Autodesk Fusion 360 part; units mm, degrees
(part 2 of 2)
sketch "Sketch26" plane through (0, 0, 10) normal (0, 0, 1) x (-1, 0, 0)
  circle A0 centre (11.42, 31.75) radius 0.762
  circle A1 centre (20.71, -12.7) radius 0.762
  circle A2 centre (23.25, 2.54) radius 0.762
  circle A3 centre (20.71, 20.32) radius 0.762
  circle A4 centre (13.96, 6.35) radius 0.762
  circle A5 centre (11.42, -13.97) radius 0.762
  circle A6 centre (8.88, -16.51) radius 0.762
  circle A7 centre (3.8, -31.75) radius 0.762
  circle A8 centre (23.25, -2.54) radius 0.762
  circle A9 centre (6.34, -34.29) radius 0.762
  circle A10 centre (3.8, -26.67) radius 0.762
  circle A11 centre (6.34, -24.13) radius 0.762
  circle A12 centre (20.71, -30.48) radius 0.762
  circle A13 centre (3.8, 3.81) radius 0.762
  circle A14 centre (3.8, 21.59) radius 0.762
  circle A15 centre (23.25, 30.48) radius 0.762
  circle A16 centre (13.96, -31.75) radius 0.762
  circle A17 centre (8.88, 19.05) radius 0.762
  circle A18 centre (11.42, 29.21) radius 0.762
  circle A19 centre (11.42, -29.21) radius 0.762
  circle A20 centre (11.42, 1.27) radius 0.762
  circle A21 centre (11.42, 3.81) radius 0.762
  circle A22 centre (3.8, -24.13) radius 0.762
  circle A23 centre (20.71, 33.02) radius 0.762
  circle A24 centre (20.71, 30.48) radius 0.762
  circle A25 centre (8.88, 21.59) radius 0.762
  circle A26 centre (6.34, -36.83) radius 0.762
  circle A27 centre (3.8, 24.13) radius 0.762
  circle A28 centre (23.25, 12.7) radius 0.762
  circle A29 centre (6.34, 26.67) radius 0.762
  circle A30 centre (13.96, 36.83) radius 0.762
  circle A31 centre (13.96, -36.83) radius 0.762
  circle A32 centre (13.96, -8.89) radius 0.762
  circle A33 centre (23.25, 0) radius 0.762
  circle A34 centre (3.8, -13.97) radius 0.762
  circle A35 centre (6.34, -6.35) radius 0.762
  circle A36 centre (11.42, -16.51) radius 0.762
  circle A37 centre (13.96, 16.51) radius 0.762
  circle A38 centre (20.71, 15.24) radius 0.762
  circle A39 centre (11.42, -19.05) radius 0.762
  circle A40 centre (20.71, -5.08) radius 0.762
  circle A41 centre (6.34, 36.83) radius 0.762
  circle A42 centre (6.34, -31.75) radius 0.762
  circle A43 centre (3.8, -21.59) radius 0.762
  circle A44 centre (13.96, 11.43) radius 0.762
  circle A45 centre (8.88, 3.81) radius 0.762
  circle A46 centre (13.96, -1.27) radius 0.762
  circle A47 centre (11.42, -34.29) radius 0.762
  circle A48 centre (23.25, -35.56) radius 0.762
  circle A49 centre (8.88, 36.83) radius 0.762
  circle A50 centre (11.42, -11.43) radius 0.762
  circle A51 centre (6.34, 8.89) radius 0.762
  circle A52 centre (3.8, -29.21) radius 0.762
  circle A53 centre (3.8, 29.21) radius 0.762
  circle A54 centre (6.34, 6.35) radius 0.762
  circle A55 centre (11.42, -1.27) radius 0.762
  circle A56 centre (6.34, 34.29) radius 0.762
  circle A57 centre (6.34, -8.89) radius 0.762
  circle A58 centre (6.34, 31.75) radius 0.762
  circle A59 centre (13.96, 13.97) radius 0.762
  circle A60 centre (8.88, 8.89) radius 0.762
  circle A61 centre (8.88, -36.83) radius 0.762
  circle A62 centre (8.88, -11.43) radius 0.762
  circle A63 centre (13.96, -29.21) radius 0.762
  circle A64 centre (20.71, 35.56) radius 0.762
  circle A65 centre (11.42, -31.75) radius 0.762
  circle A66 centre (8.88, -1.27) radius 0.762
  circle A67 centre (8.88, 13.97) radius 0.762
  circle A68 centre (23.25, 27.94) radius 0.762
  circle A69 centre (13.96, 31.75) radius 0.762
  circle A70 centre (6.34, -16.51) radius 0.762
  circle A71 centre (13.96, 26.67) radius 0.762
  circle A72 centre (6.34, -1.27) radius 0.762
  circle A73 centre (11.42, -8.89) radius 0.762
  circle A74 centre (6.34, -19.05) radius 0.762
  circle A75 centre (11.42, -3.81) radius 0.762
  circle A76 centre (8.88, 6.35) radius 0.762
  circle A77 centre (23.25, -30.48) radius 0.762
  circle A78 centre (23.25, -27.94) radius 0.762
  circle A79 centre (3.8, -3.81) radius 0.762
  circle A80 centre (11.42, 21.59) radius 0.762
  circle A81 centre (20.71, -20.32) radius 0.762
  circle A82 centre (3.8, -6.35) radius 0.762
  circle A83 centre (6.34, -3.81) radius 0.762
  circle A84 centre (13.96, -3.81) radius 0.762
  circle A85 centre (20.71, -2.54) radius 0.762
  circle A86 centre (6.34, -11.43) radius 0.762
  circle A87 centre (3.8, -16.51) radius 0.762
  circle A88 centre (23.25, 15.24) radius 0.762
  circle A89 centre (11.42, 16.51) radius 0.762
  circle A90 centre (6.34, -13.97) radius 0.762
  circle A91 centre (23.25, -10.16) radius 0.762
  circle A92 centre (3.8, 36.83) radius 0.762
  circle A93 centre (3.8, 34.29) radius 0.762
  circle A94 centre (13.96, 24.13) radius 0.762
  circle A95 centre (8.88, 29.21) radius 0.762
  circle A96 centre (11.42, 13.97) radius 0.762
  circle A97 centre (8.88, -3.81) radius 0.762
  circle A98 centre (23.25, 20.32) radius 0.762
  circle A99 centre (23.25, -33.02) radius 0.762
  circle A100 centre (23.25, -20.32) radius 0.762
  circle A101 centre (3.8, -8.89) radius 0.762
  circle A102 centre (11.42, 19.05) radius 0.762
  circle A103 centre (11.42, 26.67) radius 0.762
  circle A104 centre (20.71, 5.08) radius 0.762
  circle A105 centre (3.8, 19.05) radius 0.762
  circle A106 centre (13.96, -26.67) radius 0.762
  circle A107 centre (11.42, -6.35) radius 0.762
  circle A108 centre (8.88, -34.29) radius 0.762
  circle A109 centre (3.8, 13.97) radius 0.762
  circle A110 centre (6.34, -29.21) radius 0.762
  circle A111 centre (23.25, -5.08) radius 0.762
  circle A112 centre (20.71, 17.78) radius 0.762
  circle A113 centre (23.25, 10.16) radius 0.762
  circle A114 centre (11.42, -21.59) radius 0.762
  circle A115 centre (20.71, -17.78) radius 0.762
  circle A116 centre (11.42, -36.83) radius 0.762
  circle A117 centre (6.34, 19.05) radius 0.762
  circle A118 centre (3.8, -36.83) radius 0.762
  circle A119 centre (20.71, -25.4) radius 0.762
  circle A120 centre (3.8, 6.35) radius 0.762
  circle A121 centre (20.71, -33.02) radius 0.762
  circle A122 centre (13.96, -21.59) radius 0.762
  circle A123 centre (3.8, 1.27) radius 0.762
  circle A124 centre (6.34, 13.97) radius 0.762
  circle A125 centre (11.42, 34.29) radius 0.762
  circle A126 centre (3.8, 11.43) radius 0.762
  circle A127 centre (13.96, -34.29) radius 0.762
  circle A128 centre (8.88, 1.27) radius 0.762
  circle A129 centre (23.25, -17.78) radius 0.762
  circle A130 centre (23.25, 25.4) radius 0.762
  circle A131 centre (13.96, 29.21) radius 0.762
  circle A132 centre (8.88, 16.51) radius 0.762
  circle A133 centre (8.88, -31.75) radius 0.762
  circle A134 centre (13.96, -16.51) radius 0.762
  circle A135 centre (13.96, -11.43) radius 0.762
  circle A136 centre (8.88, 11.43) radius 0.762
  circle A137 centre (8.88, -24.13) radius 0.762
  circle A138 centre (3.8, 8.89) radius 0.762
  circle A139 centre (6.34, 3.81) radius 0.762
  circle A140 centre (20.71, -10.16) radius 0.762
  circle A141 centre (8.88, -19.05) radius 0.762
  circle A142 centre (3.8, -19.05) radius 0.762
  circle A143 centre (13.96, -24.13) radius 0.762
  circle A144 centre (8.88, -26.67) radius 0.762
  circle A145 centre (11.42, -24.13) radius 0.762
  circle A146 centre (13.96, 19.05) radius 0.762
  circle A147 centre (8.88, 34.29) radius 0.762
  circle A148 centre (6.34, -26.67) radius 0.762
  circle A149 centre (8.88, 31.75) radius 0.762
  circle A150 centre (13.96, 1.27) radius 0.762
  circle A151 centre (8.88, -21.59) radius 0.762
  circle A152 centre (13.96, 8.89) radius 0.762
  circle A153 centre (20.71, 25.4) radius 0.762
  circle A154 centre (23.25, -25.4) radius 0.762
  circle A155 centre (8.88, -8.89) radius 0.762
  circle A156 centre (3.8, 16.51) radius 0.762
  circle A157 centre (11.42, 11.43) radius 0.762
  circle A158 centre (20.71, 2.54) radius 0.762
  circle A159 centre (20.71, 10.16) radius 0.762
  circle A160 centre (23.25, -12.7) radius 0.762
  circle A161 centre (3.8, -11.43) radius 0.762
  circle A162 centre (8.88, 24.13) radius 0.762
  circle A163 centre (8.88, 26.67) radius 0.762
  circle A164 centre (8.88, -13.97) radius 0.762
  circle A165 centre (23.25, 17.78) radius 0.762
  circle A166 centre (3.8, -34.29) radius 0.762
  circle A167 centre (11.42, 36.83) radius 0.762
  circle A168 centre (20.71, -15.24) radius 0.762
  circle A169 centre (23.25, 5.08) radius 0.762
  circle A170 centre (11.42, -26.67) radius 0.762
  circle A171 centre (20.71, 12.7) radius 0.762
  circle A172 centre (13.96, -6.35) radius 0.762
  circle A173 centre (20.71, 27.94) radius 0.762
  circle A174 centre (8.88, -6.35) radius 0.762
  circle A175 centre (11.42, 24.13) radius 0.762
  circle A176 centre (8.88, -29.21) radius 0.762
  circle A177 centre (6.34, 24.13) radius 0.762
  circle A178 centre (6.34, 21.59) radius 0.762
  circle A179 centre (13.96, 21.59) radius 0.762
  circle A180 centre (3.8, 26.67) radius 0.762
  circle A181 centre (23.25, 35.56) radius 0.762
  circle A182 centre (20.71, 0) radius 0.762
  circle A183 centre (23.25, 33.02) radius 0.762
  circle A184 centre (6.34, -21.59) radius 0.762
  circle A185 centre (6.34, 29.21) radius 0.762
  circle A186 centre (11.42, 6.35) radius 0.762
  circle A187 centre (20.71, -35.56) radius 0.762
  circle A188 centre (11.42, 8.89) radius 0.762
  circle A189 centre (3.8, -1.27) radius 0.762
  circle A190 centre (6.34, 11.43) radius 0.762
  circle A191 centre (6.34, 1.27) radius 0.762
  circle A192 centre (20.71, -27.94) radius 0.762
  circle A193 centre (6.34, 16.51) radius 0.762
  circle A194 centre (13.96, -19.05) radius 0.762
  circle A195 centre (13.96, 34.29) radius 0.762
  circle A196 centre (23.25, -15.24) radius 0.762
  circle A197 centre (3.8, 31.75) radius 0.762
  circle A198 centre (13.96, -13.97) radius 0.762
  circle A199 centre (13.96, 3.81) radius 0.762
  line L0 (1.9, -40.715) -> (26.8, -40.715)
  line L1 (26.8, -40.715) -> (26.8, 40.715)
  line L2 (26.8, 40.715) -> (1.9, 40.715)
  line L3 (1.9, 40.715) -> (1.9, -40.715)
  line L4 (3.1037, 23.115) -> (-2.8963, 23.115)
  line L5 (-2.8963, 23.115) -> (-2.8963, 38.115)
  line L6 (-2.8963, 38.115) -> (3.1037, 38.115)
  line L7 (3.1037, 38.115) -> (3.1037, 23.115)
  line L8 (3.1037, 31.115) -> (-2.8963, 31.115)
  line L9 (3.1037, 30.115) -> (-2.8963, 30.115)
  line L10 (3.1037, 38.115) -> (-2.8963, 31.115) construction
  line L11 (-2.8963, 38.115) -> (3.1037, 31.115) construction
  line L12 (3.1037, 30.115) -> (-2.8963, 23.115) construction
  line L13 (-2.8963, 30.115) -> (3.1037, 23.115) construction
  circle A200 centre (0.1037, 34.615) radius 1.75
  circle A201 centre (0.1037, 26.615) radius 1.75
  line L14 (-1.5, 41.115) -> (1.5, 41.115)
  line L15 (1.5, 41.115) -> (1.5, 38.115) construction
  line L16 (1.5, 38.115) -> (-1.2925, 38.115) construction
  line L17 (-1.2925, 38.115) -> (-1.5, 41.115) construction
  dimension "d222" = 3.5
  dimension "d223" = 6
  dimension "d225" = 15
  dimension "d226" = 1
  dimension "d227" = 3
  constraint horizontal L4
  constraint vertical L5
  constraint horizontal L6
  constraint vertical L7
  constraint coincident L7 L8.start
  constraint coincident L5 L8.end
  constraint perpendicular L5 L8
  constraint coincident L7 L9.start
  constraint coincident L5 L9.end
  constraint perpendicular L5 L9
  constraint parallel L10 L12
  constraint midpoint L11 A200.centre
  constraint midpoint L13 A201.centre
  constraint equal A200 A201
  constraint coincident L14.end L15.start
  constraint perpendicular L14 L15
  constraint perpendicular L15 L16
  constraint coincident L14.start L17.end
  constraint midpoint L6 L16
  measures "d222" diameter of A201
  measures "d223" distance of L4.start L4.end
  measures "d225" distance of L4.start L6.end
  measures "d226" distance of L8 L9
  measures "d227" distance of L14 L16
extrude "Extrude19" add sketch "Sketch26" along normal blind 3.5 separate body contours A27 L7 | A27 A53 A180 L3 L4 L7 L9 | A180 L7 | L3 L4 L5 L9 | A53 L7 | L3 L5 L6 L8 | A92 A93 A197 L3 L6 L7 L8 | A197 L7 | A92 L7 | A93 L7 picked at (3.0916, 24.1999) picked at (3.0916, 26.7399) picked at (3.0916, 29.2799) picked at (3.0916, 31.8199) picked at (3.0916, 36.8999) picked at (3.0916, 34.3599) makes body 3 at (-1.7482, -34.0165, 12.3333) makes body 4 at (-1.845, -26.4408, 12.3333)
extrude "Extrude20" add sketch "Sketch26" along normal blind 5 contours A200 | A201 bodies 1 3 4
ref_plane "WorkPlane5" through (-0.1037, -26.615, 15.6) normal (0, 0, 1) x (-1, 0, 0)
sketch "Sketch27" plane through (0, 0, 15.6) normal (0, 0, 1) x (1, 0, 0)
  circle A0 centre (-0.1037, -26.615) radius 1.75
  circle A1 centre (-0.1037, -34.615) radius 1.75
  circle A2 centre (-0.1037, -34.615) radius 3.5
  circle A3 centre (-0.1037, -26.615) radius 3.5
  circle A4 centre (-0.1037, -34.615) radius 2.5
  circle A5 centre (-0.1037, -26.615) radius 2.5
  dimension "d228" = 7
  dimension "d231" = 0.75
  dimension "d232" = 0.75
  constraint concentric A1 A2
  constraint concentric A0 A3
  constraint equal A2 A3
  constraint concentric A1 A4
  constraint concentric A0 A5
  measures "d228" diameter of A3
  measures "d231" distance of A0 A5
  measures "d232" distance of A1 A4
extrude "Extrude21" cut sketch "Sketch27" along normal up to surface (6.7 mm away) contours A0 | A1 | A2 | A3 | A4 | A5 bodies 2
extrude "Extrude22" add sketch "Sketch27" along normal blind 8 separate body contours A0 | A1 | A4 | A5 makes body 5 at (2.3932, -34.7396, 20.9333) makes body 6 at (2.3932, -26.7396, 20.9333)
extrude "Extrude23" add sketch "Sketch27" along normal mid plane 0.8 from surface at 5.2 contours A2 | A3 bodies 2 5 6
sketch "case_floor" plane through (0, 0, 0) normal (0, 0, -1) x (1, 0, 0)
  line L0 (27.8, -41.715) -> (-29.3, -41.715)
  line L1 (-29.3, -41.715) -> (-29.3, 43.215)
  line L2 (-29.3, 43.215) -> (27.8, 43.215)
  line L3 (27.8, 43.215) -> (27.8, -41.715)
  line L4 (-32.3, -44.715) -> (30.8, -44.715)
  line L5 (30.8, -44.715) -> (30.8, 46.215)
  line L6 (30.8, 46.215) -> (-32.3, 46.215)
  line L7 (-32.3, 46.215) -> (-32.3, -44.715)
  line L8 (27.8, 43.215) -> (30.8, 43.215) construction
  line L9 (-29.3, 43.215) -> (-32.3, 43.215) construction
  line L10 (-29.3, -41.715) -> (-32.3, -41.715) construction
  line L11 (27.8, -41.715) -> (30.8, -41.715) construction
  circle A0 centre (33.8, 37.215) radius 6
  circle A1 centre (-35.3, 37.215) radius 6
  circle A2 centre (-35.3, -35.715) radius 6
  circle A3 centre (33.8, -35.715) radius 6
  circle A4 centre (33.8, 37.215) radius 1.65
  circle A5 centre (33.8, 37.215) radius 1.35
  circle A6 centre (33.8, -35.715) radius 1.65
  circle A7 centre (33.8, -35.715) radius 1.35
  circle A8 centre (-35.3, -35.715) radius 1.65
  circle A9 centre (-35.3, -35.715) radius 1.35
  circle A10 centre (-35.3, 37.215) radius 1.65
  circle A11 centre (-35.3, 37.215) radius 1.35
  dimension "d238" = 12
  dimension "d239" = 2.7
  dimension "d240" = 3.3
  constraint coincident L2.end L3.start
  constraint coincident L5 L8.end
  constraint perpendicular L5 L8
  constraint coincident L1.end L2.start
  constraint coincident L7 L9.end
  constraint perpendicular L7 L9
  constraint coincident L0.end L1.start
  constraint coincident L7 L10.end
  constraint perpendicular L7 L10
  constraint coincident L0.start L3.end
  constraint coincident L5 L11.end
  constraint perpendicular L5 L11
  constraint tangent L8 A0
  constraint tangent L3 A0
  constraint tangent L1 A1
  constraint tangent L9 A1
  constraint tangent L10 A2
  constraint tangent L1 A2
  constraint tangent L11 A3
  constraint tangent L3 A3
  constraint equal A0 A3
  constraint equal A2 A3
  constraint equal A1 A2
  constraint concentric A0 A4
  constraint concentric A4 A5
  constraint concentric A3 A6
  constraint concentric A3 A7
  constraint concentric A2 A8
  constraint concentric A8 A9
  constraint concentric A1 A10
  constraint concentric A1 A11
  constraint equal A7 A9
  constraint equal A5 A7
  constraint equal A5 A11
  constraint equal A4 A10
  constraint equal A4 A6
  constraint equal A6 A8
  measures "d238" diameter of A3
  measures "d239" diameter of A5
  measures "d240" diameter of A4
extrude "Extrude5" add sketch "case_floor" along normal blind 3 separate body contours L0 L1 L3 L4 L5 L7 A2 A3 | L0 L1 L2 L3 | L3 L5 A0 A3 | L5 A3 | L1 L7 A1 A2 | L7 A2 | L1 L2 L3 L5 L6 L7 A0 A1 | L5 A0 | L5 A3 | L7 A1 | L7 A2 | L5 A0 | L7 A1 makes body 7
extrude "Extrude17" add sketch "case_floor" against normal blind 7.6 contours L5 A3 | L7 A2 | L5 A0 | L7 A1 | A4 | A6 | A8 | A10 picked at (31.25, -35.715) picked at (-32.75, -35.715) picked at (31.25, 37.215) picked at (-32.75, 37.215) bodies 2
sketch "boss" plane through (0, 0, 7.6) normal (0, 0, 1) x (-1, 0, 0)
  circle A0 centre (-33.8, 37.215) radius 1.35
  arc A1 (-30.8, 42.4112) -> (-30.8, 32.0188) centre (-33.8, 37.215) ccw
  line L0 (-30.8, 32.0188) -> (-30.8, 42.4112)
  circle A2 centre (35.3, 37.215) radius 1.35
  arc A3 (32.3, 32.0188) -> (32.3, 42.4112) centre (35.3, 37.215) ccw
  line L1 (32.3, 42.4112) -> (32.3, 32.0188)
  circle A4 centre (-33.8, -35.715) radius 1.35
  arc A5 (-30.8, -30.5188) -> (-30.8, -40.9112) centre (-33.8, -35.715) ccw
  line L2 (-30.8, -40.9112) -> (-30.8, -30.5188)
  circle A6 centre (35.3, -35.715) radius 1.35
  arc A7 (32.3, -40.9112) -> (32.3, -30.5188) centre (35.3, -35.715) ccw
  line L3 (32.3, -30.5188) -> (32.3, -40.9112)
extrude "Extrude18" add sketch "boss" along normal blind 1.5 contours A0 | A1 L0 | A2 | A3 L1 | A4 | A5 L2 | A6 | A7 L3 bodies 2
sketch "leg1" plane through (0, 0, -3) normal (0, 0, -1) x (1, 0, 0)
  circle A0 centre (33.8, -35.715) radius 1.65 construction
  circle A1 centre (33.8, 37.215) radius 1.65 construction
  circle A2 centre (-35.3, 37.215) radius 1.65 construction
  circle A3 centre (-35.3, -35.715) radius 1.65 construction
  arc A4 (30.8, -40.9112) -> (30.8, -30.5188) centre (33.8, -35.715) ccw construction
  line L0 (30.8, -30.5188) -> (30.8, 32.0188) construction
  arc A5 (30.8, 32.0188) -> (30.8, 42.4112) centre (33.8, 37.215) ccw construction
  line L1 (30.8, 42.4112) -> (30.8, 46.215) construction
  line L2 (30.8, 46.215) -> (-32.3, 46.215) construction
  line L3 (-32.3, 46.215) -> (-32.3, 42.4112) construction
  arc A6 (-32.3, 42.4112) -> (-32.3, 32.0188) centre (-35.3, 37.215) ccw construction
  line L4 (-32.3, 32.0188) -> (-32.3, -30.5188) construction
  arc A7 (-32.3, -30.5188) -> (-32.3, -40.9112) centre (-35.3, -35.715) ccw construction
  line L5 (-32.3, -40.9112) -> (-32.3, -44.715) construction
  line L6 (-32.3, -44.715) -> (30.8, -44.715) construction
  line L7 (30.8, -44.715) -> (30.8, -40.9112) construction
  line L8 (-32.3, -44.715) -> (30.8, 46.215) construction
  line L9 (30.8, -44.715) -> (-32.3, 46.215) construction
  line L10 (-0.75, 0.75) -> (-0.75, -44.715) construction
  line L11 (-0.75, 0.75) -> (-0.75, 46.215) construction
  line L12 (-0.75, 0.75) -> (30.8, 0.75) construction
  line L13 (-0.75, 0.75) -> (-32.3, 0.75) construction
  circle A8 centre (-26.3, 0.75) radius 3
  circle A9 centre (-0.75, 40.215) radius 3
  circle A10 centre (24.8, 0.75) radius 3
  circle A11 centre (-0.75, -38.715) radius 3
  dimension "d243" = 6
  dimension "d244" = 6
  dimension "d245" = 6
  dimension "d246" = 6
  dimension "d247" = 6
  dimension "d248" = 6
  constraint coincident L5.end L6.start
  constraint coincident L1.end L2.start
  constraint coincident L6.end L7.start
  constraint coincident L2.end L3.start
  constraint midpoint L9 L10.start
  constraint midpoint L6 L10.end
  constraint midpoint L2 L11.end
  constraint midpoint L0 L12.end
  constraint midpoint L4 L13.end
  constraint coincident L13 A8.centre
  constraint coincident L11 A9.centre
  constraint coincident L12 A10.centre
  constraint coincident L10 A11.centre
  constraint equal A9 A10
  constraint equal A8 A11
  measures "d243" diameter of A8
  measures "d244" diameter of A9
  measures "d245" distance of L4 A8.centre
  measures "d246" distance of L12.end A10.centre
  measures "d247" distance of L11.end A9.centre
  measures "d248" distance of L10.end A11.centre
ref_plane "WorkPlane4" through (-0.75, -0.75, -6) normal (0, 0, -1) x (1, 0, 0)
sketch "leg2" plane through (0, 0, -6) normal (0, 0, -1) x (-1, 0, 0)
  circle A0 centre (-24.8, -0.75) radius 3
  circle A1 centre (26.3, -0.75) radius 3
  circle A2 centre (0.75, -40.215) radius 3
  circle A3 centre (0.75, 38.715) radius 3
  circle A4 centre (26.3, -0.75) radius 4.5
  circle A5 centre (-24.8, -0.75) radius 4.5
  circle A6 centre (0.75, 38.715) radius 4.5
  circle A7 centre (0.75, -40.215) radius 4.5
  dimension "d249" = 9
  dimension "d250" = 9
  constraint concentric A1 A4
  constraint concentric A0 A5
  constraint concentric A3 A6
  constraint concentric A2 A7
  constraint equal A4 A7
  constraint equal A5 A6
  measures "d249" diameter of A4
  measures "d250" diameter of A5
fillet "Fillet6" radius 1 20 edges at (-32.3, 40.9112, 4.55) (-32.3, 35.715, 9.1) (-32.3, 30.5188, 4.55) (-32.3, -42.4112, 4.55) (-32.3, -37.215, 9.1) (-32.3, -32.0188, 4.55) (30.8, 40.9112, 4.55) (30.8, 35.715, 9.1) (30.8, 30.5188, 4.55) (30.8, -42.4112, 4.55) (30.8, -37.215, 9.1) (30.8, -32.0188, 4.55) (30.8, -32.0188, -1.5) (30.8, -42.4112, -1.5) (30.8, 30.5188, -1.5) (30.8, 40.9112, -1.5) (-32.3, 40.9112, -1.5) (-32.3, 30.5188, -1.5) (-32.3, -42.4112, -1.5) (-32.3, -32.0188, -1.5) on bodies 2 7
loft "Loft5" add profiles "leg1", "leg2" section 1 contours A8 section 2 contours A1 | A4 bodies 7
loft "Loft6" add profiles "leg1", "leg2" section 1 contours A11 section 2 contours A3 | A6 bodies 7
loft "Loft7" add profiles "leg1", "leg2" section 1 contours A10 section 2 contours A0 | A5 bodies 7
loft "Loft8" add profiles "leg1", "leg2" section 1 contours A9 section 2 contours A2 | A7 bodies 7
equation "d1 = board_width"
equation "d2 = board_length"
equation "d5 = d2 / 2"
equation "d7 = d1 / 2"
equation "d8 = board_height"
equation "ravine_width = ravine_wdith"
equation "pin_spacing = 0.1 in"
equation "d35 = pin_spacing * 4"
equation "d36 = -pin_spacing * 14"
equation "d40 = pin_spacing"
equation "d41 = 2 * pin_spacing"
equation "d45 = 12 * pin_spacing"
equation "board_width = 54.4 mm"
equation "board_length = 82.23 mm"
equation "board_height = 10 mm"
equation "d66 = -board_height - tolerance - rasberry_pi_height - 3 mm"
equation "d68 = case_width"
equation "case_width = 3 mm"
equation "ravine_wdith = 3 mm"
equation "d85 = ravine_wdith"
equation "d87 = ravine_wdith"
equation "d90 = ravine_wdith"
equation "d94 = ravine_wdith"
equation "tolerance = 0.6 mm"
equation "peg_height = 5 mm"
equation "rasberry_pi_height = 5.7 mm"
equation "d101 = rasberry_pi_length"
equation "rasberry_pi_length = 58 mm"
equation "d106 = case_width"
equation "d155 = -7.00 mm - tolerance"
equation "d199 = tolerance"
equation "d200 = tolerance"
equation "d201 = tolerance"
equation "d202 = tolerance"
equation "d203 = case_width"
equation "d204 = case_width"
equation "d205 = case_width"
equation "d206 = case_width"
equation "d221 = tolerance"
named bodies: "breadboard_body", "case_base", "case_floor", "button", "button2"
